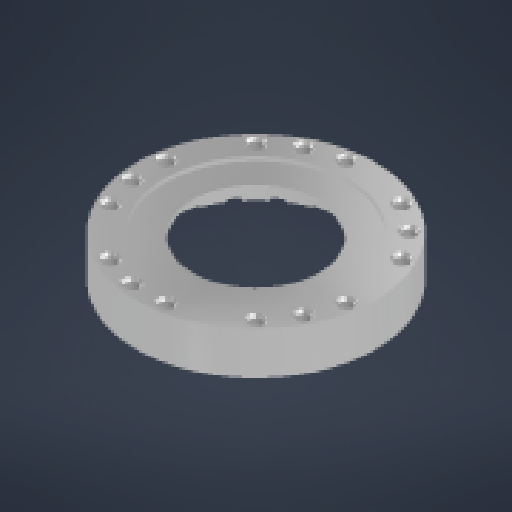
# Autodesk Inventor part: Case_Taped_GB
Saved by Autodesk Inventor 2024.2 (Build 282272000, 272)
## iProperties
Created: 2026-01-04
Part Number: Case_Taped_GB
Material: Aluminum 6061
Document SubType Name: Modeling
Designer: 4aida
Density: 2.7 g/cm^3
Appearance: Aluminum - Flat
Author: 4aida
Autodesk Inventor part; units mm, degrees
ref_plane "YZ Plane" through (0, 0, 0) normal (1, 0, 0) x (0, 1, 0)
ref_plane "XZ Plane" through (0, 0, 0) normal (0, 1, 0) x (-1, 0, 0)
ref_plane "XY Plane" through (0, 0, 0) normal (0, 0, 1) x (1, 0, 0)
sketch "Sketch1" plane through (0, 0, 0) normal (0, 0, 1) x (1, 0, 0)
  line L0 (0, 7.6) -> (0, -7.6)
  line L1 (42.5, -7.6) -> (42.5, 7.6)
  line L2 (42.5, 7.6) -> (22.5, 7.6)
  line L3 (22.5, 7.6) -> (22.5, 4.6)
  line L4 (22.5, 4.6) -> (29, 4.6)
  line L5 (29, 4.6) -> (29, -2.4)
  line L6 (29, -2.4) -> (35, -2.4)
  line L7 (35, -2.4) -> (35, -7.6)
  line L8 (35, -7.6) -> (42.5, -7.6)
  point P0 (0, 0)
  point P1 (0, 0)
  dimension "d0" = 58
  dimension "d1" = 7
  dimension "d2" = 45
  dimension "d3" = 3
  dimension "d4" = 5.2
  dimension "d5" = 70
  dimension "d6" = 85
  constraints: 18 end point, 7 perpendicular, 2 horizontal alignment, 2 vertical, 1 coincident, 1 midpoint
  measures "d0" diameter of L5 L0
  measures "d1" distance of L4.end L5.end
  measures "d2" diameter of L3 L0
  measures "d3" distance of L2.end L3.end
  measures "d4" distance between parallel lines of L8 L6
  measures "d5" diameter of L7 L0
  measures "d6" diameter of L1 L0
revolve "Revolution1" add sketch "Sketch1" angle 360 about axis through (0, 7.6, 0) along (0, -1, 0)
sketch "Sketch2" plane through (0, -7.6, 0) normal (0, -1, 0) x (1, 0, 0)
  point P0 (0, 0)
  point P1 (-35, 0)
  dimension "d8" = 35
  constraints: 1 horizontal alignment
  measures "d8" distance of point (0, 0) point (-35, 0)
hole "Hole1" at (-35, -7.6, 0) direction (0, 1, 0) diameter 4 depth 10 tip angle 118
pattern_circular "Circular Pattern1" count 20 over 360 about axis through (0, -5, 0) along (0, -1, 0) of "Hole1"
sketch "Sketch5" plane through (0, -7.6, 0) normal (0, -1, 0) x (1, 0, 0)
  line L0 (0, 0) -> (38.5198, -6.1009)
  circle A0 centre (38.5198, -6.1009) radius 3.5
  circle A1 centre (0, 0) radius 42.5 projected
  arc A2 (34.9429, 1.9992) -> (34.9429, -1.9992) centre (35, 0) ccw projected
  line L1 (0, 0) -> (35, 0)
  dimension "d41" = 7
  dimension "d42" = 9
  constraints: 4 end point, 1 centre point, 1 coincident, 1 horizontal, 1 tangent
  measures "d41" diameter of A0
  measures "d42" angle of L0 L1
hole "Hole3" at (38.5198, -7.6, -6.1009) direction (0, 1, 0) diameter 3.242 depth 11.8 tip angle 118 countersink diameter 4 countersink angle 90 thread size "M4x0.7" class "6H" standard "ANSI Metric M Profile"
pattern_circular "Circular Pattern3" count 5 over 360 about axis through (0, 6.1, 0) along (0, -1, 0) of "Hole3"
sketch "Sketch6" plane through (0, 7.6, 0) normal (0, 1, 0) x (1, 0, 0)
  circle A0 centre (0, 0) radius 42.5 projected
  line L0 (-38.026, -6.0227) -> (0, 0)
  line L1 (0, 0) -> (-42.5, 0)
  point P0 (0, 0)
  point P1 (-34.3038, -17.4786)
  point P2 (-27.2236, -27.2236)
  point P3 (-17.4786, -34.3038)
  point P4 (-6.0227, -38.026)
  point P5 (6.0227, -38.026)
  point P6 (17.4786, -34.3038)
  point P7 (27.2236, -27.2236)
  point P8 (34.3038, -17.4786)
  point P9 (38.026, -6.0227)
  point P10 (38.026, 6.0227)
  point P11 (34.3038, 17.4786)
  point P12 (27.2236, 27.2236)
  point P13 (17.4786, 34.3038)
  point P14 (6.0227, 38.026)
  point P15 (-6.0227, 38.026)
  point P16 (-17.4786, 34.3038)
  point P17 (-27.2236, 27.2236)
  point P18 (-34.3038, 17.4786)
  point P19 (-38.026, 6.0227)
  dimension "d53" = 38.5
  dimension "d54" = 9
  dimension "d57" = 360
  constraints: 4 end point, 1 horizontal, 1 horizontal alignment, 22 other
  measures "d53" distance of point (0, 0) L0.start
  measures "d54" angle of L1 L0
hole "Hole4" at (-38.026, 7.6, 6.0227) at (-34.3038, 7.6, 17.4786) at (-17.4786, 7.6, 34.3038) at (-6.0227, 7.6, 38.026) at (6.0227, 7.6, 38.026) at (27.2236, 7.6, 27.2236) at (34.3038, 7.6, 17.4786) at (38.026, 7.6, 6.0227) at (34.3038, 7.6, -17.4786) at (27.2236, 7.6, -27.2236) at (17.4786, 7.6, -34.3038) at (-6.0227, 7.6, -38.026) at (-17.4786, 7.6, -34.3038) at (-27.2236, 7.6, -27.2236) at (-38.026, 7.6, -6.0227) direction (0, -1, 0) diameter 4.134 depth 12 tip angle 118 countersink diameter 6 countersink angle 90 thread size "M5x0.8" class "6H" standard "ANSI Metric M Profile"
sketch "Sketch7" plane through (0, 7.6, 0) normal (0, 1, 0) x (1, 0, 0)
  circle A0 centre (0, 0) radius 32.6
  point P0 (0, 0)
  dimension "d66" = 65.2
  constraints: 1 centre point, 1 coincident
  measures "d66" diameter of A0
extrude "Extrusion2" cut sketch "Sketch7" against normal blind 1.5
body "Solid1"
